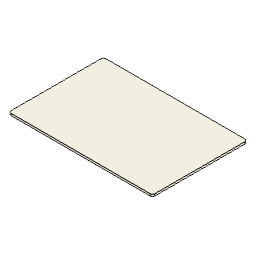
bottom1 (Autodesk Fusion 360 design; units mm, degrees)
part number: 2025-09-30-18-36-47-433
Autodesk Fusion 360 part; units mm, degrees
sketch "Sketch1" plane through (0, 0, 0) normal (0, 0, 1) x (1, 0, 0)
  line L0 (5, 0) -> (306, 0)
  line L1 (311, 5) -> (311, 200)
  line L2 (306, 205) -> (5, 205)
  line L3 (0, 200) -> (0, 5)
  arc A0 (5, 205) -> (0, 200) centre (5, 200) ccw
  arc A1 (311, 200) -> (306, 205) centre (306, 200) ccw
  arc A2 (0, 5) -> (5, 0) centre (5, 5) ccw
  arc A3 (306, 0) -> (311, 5) centre (306, 5) ccw
  dimension "d1" = 311
  dimension "d2" = 205
  dimension "d3" = 5
  dimension "d4" = 5
  dimension "d5" = 5
  dimension "d6" = 5
  constraint horizontal L0
  constraint vertical L1
  constraint horizontal L2
  constraint vertical L3
  constraint tangent L2 A0
  constraint tangent L3 A0
  constraint tangent L1 A1
  constraint tangent L2 A1
  constraint tangent L0 A2
  constraint tangent L3 A2
  constraint tangent L0 A3
  constraint tangent L1 A3
  measures "d1" distance of L1 L3
  measures "d2" distance of L0 L2
  measures "d3" radius of A0
  measures "d4" radius of A1
  measures "d5" radius of A2
  measures "d6" radius of A3
extrude "Extrude1" add sketch "Sketch1" along normal blind 4.5
sketch "Sketch2" plane through (0, 0, 0) normal (0, 0, 1) x (1, 0, 0)
  circle A0 centre (20, 20) radius 7.5
  line L0 (0, 200) -> (0, 5)
  line L1 (5, 0) -> (306, 0)
  circle A1 centre (291, 20) radius 7.5
  line L2 (311, 5) -> (311, 200)
  circle A2 centre (20, 185) radius 7.5
  line L3 (306, 205) -> (5, 205)
  circle A3 centre (291, 185) radius 7.5
  dimension "d9" = 15
  dimension "d10" = 20
  dimension "d11" = 20
  dimension "d12" = 15
  dimension "d13" = 20
  dimension "d14" = 20
  dimension "d15" = 15
  dimension "d16" = 20
  dimension "d17" = 20
  dimension "d18" = 15
  dimension "d19" = 20
  dimension "d20" = 20
  measures "d9" diameter of A0
  measures "d10" distance of A0.centre L0
  measures "d11" distance of A0.centre L1
  measures "d12" diameter of A1
  measures "d13" distance of A1.centre L2
  measures "d14" distance of L1 A1.centre
  measures "d15" diameter of A2
  measures "d16" distance of A2.centre L3
  measures "d17" distance of L0 A2.centre
  measures "d18" diameter of A3
  measures "d19" distance of L3 A3.centre
  measures "d20" distance of L2 A3.centre
extrude "Extrude2" add sketch "Sketch2" against normal blind 2.5
